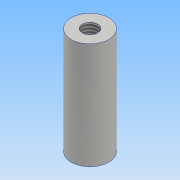
# Autodesk Inventor part: Top_Separator Weight
Saved by Autodesk Inventor 2018.1 (Build 221171000, 171)
## iProperties
Created: 2019-02-11
Part Number: Top_Separator Weight
Material: Aluminum 6061
Document SubType Name: Modeling
Designer: James
Density: 2.7 g/cm^3
Appearance: Aluminum - Flat
Author: James
Autodesk Inventor part; units mm, degrees
ref_plane "YZ Plane" through (0, 0, 0) normal (1, 0, 0) x (0, 1, 0)
ref_plane "XZ Plane" through (0, 0, 0) normal (0, 1, 0) x (-1, 0, 0)
ref_plane "XY Plane" through (0, 0, 0) normal (0, 0, 1) x (1, 0, 0)
sketch "Sketch1" plane through (0, 0, 0) normal (0, 0, 1) x (1, 0, 0)
  circle A0 centre (0, 0) radius 3
  dimension "d0" = 6
  constraints: 1 centre point, 1 coincident
  measures "d0" diameter of A0
extrude "Extrusion1" add sketch "Sketch1" along normal blind 17
sketch "Sketch2" plane through (0, 0, 17) normal (0, 0, 1) x (1, 0, 0)
  point P0 (0, 0)
  point P1 (0, 0)
  constraints: 1 coincident
hole "Hole1" at (0, 0, 17) direction (0, 0, -1) diameter 2.459 end through all thread size "M3x0.5" class "6H" standard "ANSI Metric M Profile"
sketch "Sketch3" plane through (0, 0, 0) normal (0, 1, 0) x (-1, 0, 0)
  line L0 (3, 0) -> (3, 17) projected
  line L1 (3, 17) -> (2.5, 17)
  line L2 (2.5, 17) -> (2.5, 13)
  line L3 (2.5, 13) -> (3, 13)
  line L4 (3, 13) -> (3, 17)
  line L5 (3, 17) -> (-3, 17) projected
  line L6 (-3, 17) -> (-2.5, 17)
  line L7 (-2.5, 17) -> (-2.5, 13)
  line L8 (-2.5, 13) -> (-3, 13)
  line L9 (-3, 13) -> (-3, 17)
  point P0 (0, 0)
  dimension "d10" = 0.5
  dimension "d11" = 5
  dimension "d12" = 0.5
  dimension "d13" = 4
  constraints: 16 end point, 4 parallel, 2 horizontal, 2 perpendicular, 2 point on line
  measures "d10" distance between parallel lines of L0 L2
  measures "d11" distance between parallel lines of L7 L2
  measures "d12" distance between parallel lines of L7 L9
  measures "d13" distance of L6.end L7.end
extrude "Extrusion2" [suppressed]
equation "\"d10\" = d12"
body "Solid1"
